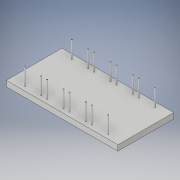
# Autodesk Inventor part: fuselage
Saved by Autodesk Inventor 2018 (Build 220112000, 112)
## iProperties
Created: 2017-12-28
Part Number: fuselage
Material: Generic
Document SubType Name: Modeling
Designer: BB-8
Density: 1 g/cm^3
Appearance: Default
Author: BB-8
Autodesk Inventor part; units mm, degrees
ref_plane "YZ Plane" through (0, 0, 0) normal (1, 0, 0) x (0, 1, 0)
ref_plane "XZ Plane" through (0, 0, 0) normal (0, 1, 0) x (-1, 0, 0)
ref_plane "XY Plane" through (0, 0, 0) normal (0, 0, 1) x (1, 0, 0)
sketch "Sketch3" plane through (0, 0, 0) normal (0, 1, 0) x (-1, 0, 0)
  line L0 (0, 0) -> (200, 0)
  line L1 (200, 0) -> (200, -100)
  line L2 (200, -100) -> (0, -100)
  line L3 (0, -100) -> (0, 0)
  circle A0 centre (54.65, -7.9) radius 1
  circle A1 centre (25.35, -7.9) radius 1
  circle A2 centre (54.65, -92.1) radius 1
  circle A3 centre (25.35, -92.1) radius 1
  circle A4 centre (145.35, -7.9) radius 1
  circle A5 centre (174.65, -7.9) radius 1
  circle A6 centre (145.35, -92.1) radius 1
  circle A7 centre (174.65, -92.1) radius 1
  circle A8 centre (94.65, -7.9) radius 1
  circle A9 centre (65.35, -7.9) radius 1
  circle A10 centre (94.65, -92.1) radius 1
  circle A11 centre (65.35, -92.1) radius 1
  circle A12 centre (105.35, -7.9) radius 1
  circle A13 centre (134.65, -7.9) radius 1
  circle A14 centre (134.65, -92.1) radius 1
  circle A15 centre (105.35, -92.1) radius 1
  dimension "d5" = 200
  dimension "d6" = 100
  dimension "d8" = 2
  dimension "d9" = 2
  constraints: 16 centre point, 8 end point, 2 coincident, 2 parallel, 1 horizontal, 1 perpendicular
  measures "d5" distance of L1.end L2.end
  measures "d6" distance of L0.end L1.end
  measures "d8" diameter of A0
  measures "d9" diameter of A8
extrude "Extrusion2" add sketch "Sketch3" along normal blind 30 contours A1
extrude "Extrusion3" add sketch "Sketch3" along normal blind 30 contours A0 | A2 | A3 | A4 | A5 | A6 | A7 | A8 | A9 | A10 | A11 | A12 | A13 | A14 | A15
extrude "Extrusion4" add sketch "Sketch3" against normal blind 10
body "Solid2"
